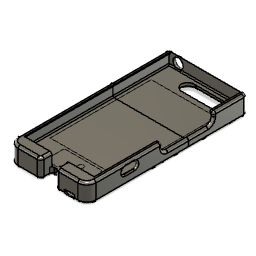
CoverMk5 v70 (Autodesk Fusion 360 design; units mm, degrees)
part number: BottomLid
Autodesk Fusion 360 part; units mm, degrees
(part 1 of 2)
sketch "Sketch1" plane through (0, 0, 0) normal (0, 1, 0) x (1, 0, 0) in component "BottomPart"
  line L0 (0, 0) -> (69, 0)
  line L1 (0, 0) -> (0, -90)
  line L2 (0, -90) -> (69, -90)
  line L3 (69, -90) -> (69, 0)
  line L4 (69, 0) -> (0, 0)
  line L5 (0, 0) -> (0, -90)
  dimension "d1" = 69
  dimension "d2" = 90
  constraint coincident L0.start L1.start
  constraint horizontal L0
  constraint perpendicular L0 L1
  constraint horizontal L2
  constraint vertical L3
  constraint horizontal L4
  constraint vertical L5
  measures "d1" distance of L0.start L0.end
  measures "d2" distance of L0.start L1.end
extrude "Extrude1" add sketch "Sketch1" along normal blind 0.5 makes body 1 in component "BottomPart"
sketch "Sketch2" plane through (0, 0.5, 0) normal (0, 1, 0) x (-1, 0, 0) in component "BottomPart"
  line L0 (0, 0) -> (0, 90)
  line L1 (0, 90) -> (-69, 90)
  line L2 (-69, 90) -> (-69, 0)
  line L3 (-69, 0) -> (0, 0)
  line L4 (0, 90) -> (-28, 90)
  line L5 (-69, 90) -> (-41, 90)
  line L6 (-41, 90) -> (-41, 80)
  line L7 (-41, 80) -> (-28, 80)
  line L8 (-28, 80) -> (-28, 90)
  line L9 (-28, 90) -> (-41, 90)
  line L10 (-41, 90) -> (-41, 80)
  dimension "d5" = 28
  dimension "d6" = 28
  dimension "d7" = 10
  constraint coincident L0.end L1.start
  constraint perpendicular L0 L4
  constraint coincident L1.end L2.start
  constraint perpendicular L2 L5
  constraint perpendicular L5 L6
  constraint horizontal L7
  constraint vertical L8
  constraint horizontal L9
  constraint vertical L10
  measures "d5" distance of L0.end L4.end
  measures "d6" distance of L1.end L5.end
  measures "d7" distance of L5.end L6.end
extrude "Extrude2" cut sketch "Sketch2" against normal blind 2 contours L1 L6 L7 L8 L9 L10 bodies 1 in component "BottomPart"
sketch "Sketch3" plane through (0, 0.5, 0) normal (0, 1, 0) x (-1, 0, 0) in component "BottomPart"
  line L0 (-41, 80) -> (-41, 90)
  line L1 (-41, 90) -> (-69, 90)
  line L2 (-69, 90) -> (-69, 0)
  line L3 (-69, 0) -> (0, 0)
  line L4 (0, 0) -> (0, 90)
  line L5 (0, 90) -> (-28, 90)
  line L6 (-28, 90) -> (-28, 80)
  line L7 (-28, 80) -> (-41, 80)
  line L8 (0, 0) -> (-2, 0)
  line L9 (-28, 80) -> (0, 80)
  line L10 (-2, 0) -> (-2, 80)
  line L11 (-41, 80) -> (-69, 80)
  line L12 (-69, 0) -> (-67, 0)
  line L13 (-67, 0) -> (-67, 80)
  dimension "d10" = 2
  dimension "d11" = 2
  constraint coincident L3.end L4.start
  constraint perpendicular L4 L8
  constraint coincident L6.end L7.start
  constraint coincident L4 L9.end
  constraint perpendicular L4 L9
  constraint coincident L9 L10.end
  constraint perpendicular L9 L10
  constraint coincident L0.start L7.end
  constraint coincident L2 L11.end
  constraint perpendicular L2 L11
  constraint coincident L2.end L3.start
  constraint perpendicular L2 L12
  constraint coincident L11 L13.end
  constraint perpendicular L11 L13
  measures "d10" distance of L3.end L8.end
  measures "d11" distance of L2.end L12.end
extrude "Extrude3" add sketch "Sketch3" along normal blind 10.5 contours L0 L1 L2 L11 | L4 L5 L6 L9 | L2 L3 L11 L12 L13 | L3 L4 L8 L9 L10 bodies 1 in component "BottomPart"
extrude "Extrude4" add 1 faces at (32.3333, 0, 26.6667) along direction (0, -1, 0) blind 4 on bodies 1 bodies 1 in component "BottomPart"
sketch "Sketch13" plane through (0, -4, 0) normal (0, -1, 0) x (1, 0, 0) in component "BottomPart"
  line L0 (41, 90) -> (41, 80)
  line L1 (41, 80) -> (28, 80)
  line L2 (28, 80) -> (28, 90)
  line L3 (28, 90) -> (0, 90)
  line L4 (0, 90) -> (0, 0)
  line L5 (0, 0) -> (69, 0)
  line L6 (69, 0) -> (69, 90)
  line L7 (69, 90) -> (41, 90)
  line L8 (0, 90) -> (2, 90)
  line L9 (2, 90) -> (2, 88)
  line L10 (2, 88) -> (0, 88)
  line L11 (0, 88) -> (0, 90)
  line L12 (28, 90) -> (26, 90)
  line L13 (26, 90) -> (26, 88)
  line L14 (26, 88) -> (28, 88)
  line L15 (28, 88) -> (28, 90)
  line L16 (28, 80) -> (26, 80)
  line L17 (26, 80) -> (26, 78)
  line L18 (26, 78) -> (28, 78)
  line L19 (28, 78) -> (28, 80)
  line L20 (41, 80) -> (43, 80)
  line L21 (43, 80) -> (43, 78)
  line L22 (43, 78) -> (41, 78)
  line L23 (41, 78) -> (41, 80)
  line L24 (41, 90) -> (43, 90)
  line L25 (43, 90) -> (43, 88)
  line L26 (43, 88) -> (41, 88)
  line L27 (41, 88) -> (41, 90)
  line L28 (69, 90) -> (67, 90)
  line L29 (67, 90) -> (67, 88)
  line L30 (67, 88) -> (69, 88)
  line L31 (69, 88) -> (69, 90)
  line L32 (69, 0) -> (67, 0)
  line L33 (0, 0) -> (2, 0)
  line L34 (2, 0) -> (2, 88)
  line L35 (26, 88) -> (2, 88)
  line L36 (26, 88) -> (26, 80)
  line L37 (28, 78) -> (41, 78)
  line L38 (43, 80) -> (43, 88)
  line L39 (43, 88) -> (67, 88)
  line L40 (67, 88) -> (67, 0)
  dimension "d181" = 2
  dimension "d182" = 2
  dimension "d183" = 2
  dimension "d184" = 2
  dimension "d185" = 2
  dimension "d186" = 2
  dimension "d187" = 2
  dimension "d188" = 2
  dimension "d189" = 2
  dimension "d190" = 2
  dimension "d191" = 2
  dimension "d192" = 2
  dimension "d193" = 2
  dimension "d194" = 2
  constraint horizontal L8
  constraint vertical L9
  constraint horizontal L10
  constraint vertical L11
  constraint coincident L3.end L4.start
  constraint horizontal L12
  constraint vertical L13
  constraint horizontal L14
  constraint vertical L15
  constraint coincident L2.end L3.start
  constraint horizontal L16
  constraint vertical L17
  constraint horizontal L18
  constraint vertical L19
  constraint coincident L1.end L2.start
  constraint horizontal L20
  constraint vertical L21
  constraint horizontal L22
  constraint vertical L23
  constraint coincident L0.end L1.start
  constraint horizontal L24
  constraint vertical L25
  constraint horizontal L26
  constraint vertical L27
  constraint coincident L0.start L7.end
  constraint horizontal L28
  constraint vertical L29
  constraint horizontal L30
  constraint vertical L31
  constraint coincident L6.end L7.start
  constraint coincident L5.end L6.start
  constraint perpendicular L6 L32
  constraint coincident L4.end L5.start
  constraint perpendicular L4 L33
  measures "d181" distance of L3.end L8.end
  measures "d182" distance of L3.end L10.end
  measures "d183" distance of L2.end L12.end
  measures "d184" distance of L2.end L14.end
  measures "d185" distance of L1.end L16.end
  measures "d186" distance of L1.end L18.end
  measures "d187" distance of L0.end L20.end
  measures "d188" distance of L0.end L22.end
  measures "d189" distance of L0.start L24.end
  measures "d190" distance of L0.start L26.end
  measures "d191" distance of L6.end L28.end
  measures "d192" distance of L6.end L30.end
  measures "d193" distance of L5.end L32.end
  measures "d194" distance of L4.end L33.end
extrude "Extrude19" cut sketch "Sketch13" against normal blind 4 contours L5 L17 L18 L21 L22 L34 L35 L36 L37 L38 L39 L40 bodies 1 in component "BottomPart"
sketch "Sketch4" plane through (0, 0, 0) normal (0, -1, 0) x (1, 0, 0) in component "BottomPart"
  line L0 (2, 88) -> (2, 2)
  line L1 (2, 2) -> (67, 2)
  line L2 (67, 2) -> (67, 88)
  line L3 (67, 88) -> (43, 88)
  line L4 (43, 88) -> (43, 78)
  line L5 (43, 78) -> (26, 78)
  line L6 (26, 78) -> (26, 88)
  line L7 (26, 88) -> (2, 88)
  line L8 (67, 88) -> (66, 88)
  line L9 (66, 88) -> (66, 82)
  line L10 (66, 82) -> (67, 82)
  line L11 (67, 82) -> (67, 88)
  circle A0 centre (66, 82) radius 0.95
  line L12 (66, 82) -> (64, 82)
  line L13 (64, 82) -> (64, 88)
  line L14 (64, 82) -> (67, 82)
  line L15 (67, 82) -> (67, 79)
  line L16 (67, 79) -> (64, 79)
  line L17 (64, 79) -> (64, 82)
  line L18 (43, 78) -> (39, 78)
  line L19 (39, 78) -> (39, 72)
  line L20 (39, 72) -> (43, 72)
  line L21 (43, 72) -> (43, 78)
  line L22 (41, 78) -> (41, 72)
  circle A1 centre (41, 75) radius 0.95
  line L23 (43, 88) -> (43, 78)
  line L24 (43, 78) -> (26, 78)
  line L25 (26, 78) -> (26, 88)
  line L26 (26, 88) -> (2, 88)
  line L27 (2, 88) -> (2, 0)
  line L28 (2, 0) -> (67, 0)
  line L29 (67, 0) -> (67, 88)
  line L30 (67, 88) -> (43, 88)
  dimension "d19" = 1
  dimension "d20" = 6
  dimension "d21" = 1.9
  dimension "d22" = 2
  dimension "d23" = 3
  dimension "d24" = 4
  dimension "d25" = 6
  dimension "d26" = 1.9
  constraint horizontal L8
  constraint vertical L9
  constraint horizontal L10
  constraint vertical L11
  constraint coincident L2.end L3.start
  constraint coincident L9.end L10.start
  constraint perpendicular L9 L12
  constraint coincident L3 L13.end
  constraint perpendicular L3 L13
  constraint horizontal L14
  constraint vertical L15
  constraint horizontal L16
  constraint vertical L17
  constraint horizontal L18
  constraint vertical L19
  constraint horizontal L20
  constraint vertical L21
  constraint coincident L4.end L5.start
  constraint midpoint L18 L22.start
  constraint midpoint L20 L22.end
  constraint midpoint L22 A1.centre
  measures "d19" distance of L2.end L8.end
  measures "d20" distance of L2.end L10.end
  measures "d21" diameter of A0
  measures "d22" distance of L9.end L12.end
  measures "d23" distance of L12.end L16.end
  measures "d24" distance of L4.end L18.end
  measures "d25" distance of L4.end L20.end
  measures "d26" diameter of A1
extrude "Extrude6" add sketch "Sketch4" along normal blind 4 contours L2 L10 A0 L12 L14 L15 L16 L17 L29 | L5 L18 L19 L20 L22 A1 L24 | L2 L3 L8 L9 L10 L11 A0 L14 L29 L30 | L5 L18 L20 L21 L22 A1 L24 | L3 L9 A0 L12 L13 L14 L30 bodies 1 in component "BottomPart"
sketch "Sketch5" plane through (0, -4, 0) normal (0, -1, 0) x (1, 0, 0) in component "BottomPart"
  line L0 (34.5, 80) -> (30.5, 80)
  line L1 (30.5, 80) -> (38.5, 80)
  line L2 (38.5, 80) -> (38.5, 78)
  line L3 (38.5, 78) -> (30.5, 78)
  line L4 (30.5, 78) -> (30.5, 80)
  line L5 (67, 79) -> (67, 0)
  line L6 (67, 0) -> (69, 0)
  line L7 (69, 0) -> (69, 90)
  line L8 (69, 90) -> (41, 90)
  line L9 (41, 90) -> (41, 80)
  line L10 (41, 80) -> (28, 80)
  line L11 (28, 80) -> (28, 90)
  line L12 (28, 90) -> (0, 90)
  line L13 (0, 90) -> (0, 0)
  line L14 (0, 0) -> (2, 0)
  line L15 (2, 0) -> (2, 88)
  line L16 (2, 88) -> (26, 88)
  line L17 (26, 88) -> (26, 78)
  line L18 (26, 78) -> (39, 78)
  line L19 (43, 72) -> (43, 88)
  line L20 (43, 88) -> (64, 88)
  circle A0 centre (41, 75) radius 0.95
  line L21 (39, 78) -> (39, 72)
  line L22 (39, 72) -> (43, 72)
  line L23 (64, 88) -> (64, 79)
  line L24 (64, 79) -> (67, 79)
  circle A1 centre (66, 82) radius 0.95
  dimension "d29" = 4
  dimension "d30" = 8
  constraint horizontal L1
  constraint vertical L2
  constraint horizontal L3
  constraint vertical L4
  measures "d29" distance of L0.start L0.end
  measures "d30" distance of L0.end L1.end
extrude "Extrude7" cut sketch "Sketch5" against normal blind 2.5 contours L0 L1 L2 L3 L4 L10 L18 bodies 1 in component "BottomPart"
sketch "Sketch6" plane through (0, 0, 0) normal (0, -1, 0) x (1, 0, 0) in component "BottomPart"
  line L0 (43, 88) -> (64, 88)
  line L1 (64, 88) -> (64, 61)
  line L2 (64, 61) -> (43, 61)
  line L3 (43, 61) -> (43, 88)
  line L4 (64, 61) -> (67, 61)
  line L5 (64, 61) -> (64, 60)
  line L6 (64, 60) -> (2, 60)
  line L7 (2, 60) -> (2, 61)
  line L8 (2, 61) -> (64, 61)
  line L9 (64, 61) -> (64, 60)
  line L10 (43, 72) -> (39, 72)
  line L11 (39, 72) -> (39, 65)
  line L12 (39, 65) -> (43, 65)
  line L13 (43, 65) -> (43, 72)
  line L14 (26, 78) -> (20, 78)
  line L15 (20, 78) -> (20, 61)
  line L16 (64, 61) -> (67, 61)
  line L17 (67, 61) -> (67, 65)
  line L18 (67, 65) -> (64, 65)
  line L19 (64, 65) -> (64, 61)
  line L20 (30.5, 78) -> (38.5, 78)
  line L21 (38.5, 78) -> (38.5, 80)
  line L22 (38.5, 80) -> (30.5, 80)
  line L23 (30.5, 80) -> (30.5, 78)
  line L24 (39, 72) -> (39, 78)
  line L25 (39, 78) -> (26, 78)
  line L26 (26, 78) -> (26, 88)
  line L27 (26, 88) -> (2, 88)
  line L28 (2, 88) -> (2, 0)
  line L29 (2, 0) -> (67, 0)
  line L30 (67, 0) -> (67, 79)
  line L31 (67, 79) -> (64, 79)
  line L32 (64, 79) -> (64, 88)
  line L33 (64, 88) -> (43, 88)
  line L34 (43, 88) -> (43, 72)
  line L35 (43, 72) -> (39, 72)
  dimension "d33" = 21
  dimension "d34" = 27
  dimension "d35" = 1
  dimension "d36" = 1
  dimension "d37" = 4
  dimension "d38" = 7
  dimension "d39" = 6
  dimension "d42" = 4
  constraint horizontal L0
  constraint vertical L1
  constraint horizontal L2
  constraint vertical L3
  constraint perpendicular L2 L5
  constraint horizontal L6
  constraint vertical L7
  constraint horizontal L8
  constraint vertical L9
  constraint horizontal L10
  constraint vertical L11
  constraint horizontal L12
  constraint vertical L13
  constraint coincident L8 L15.end
  constraint perpendicular L8 L15
  constraint horizontal L16
  constraint vertical L17
  constraint horizontal L18
  constraint vertical L19
  measures "d33" distance of L0.start L0.end
  measures "d34" distance of L0.start L2.end
  measures "d35" distance of L1.end L5.end
  measures "d36" distance of L5.end L1.end
  measures "d37" distance of L10.start L10.end
  measures "d38" distance of L10.start L12.end
  measures "d39" distance of L14.start L14.end
  measures "d42" distance of L1.end L18.end
extrude "Extrude8" add sketch "Sketch6" along normal blind 4 contours L3 L10 L11 L12 L13 L35 | L1 L18 L30 L31 | L2 L5 L6 L7 L8 L9 L28 | L8 L14 L15 L26 L27 L28 bodies 1 in component "BottomPart"
sketch "Sketch7" plane through (0, -4, 0) normal (0, -1, 0) x (1, 0, 0) in component "BottomPart"
  line L0 (0, 90) -> (3, 90)
  line L1 (3, 90) -> (3, 82)
  line L2 (3, 82) -> (0, 82)
  line L3 (0, 82) -> (0, 90)
  circle A0 centre (3, 82) radius 0.95
  line L4 (41, 80) -> (38.5, 80)
  line L5 (69, 90) -> (41, 90)
  line L6 (67, 0) -> (69, 0)
  line L7 (38.5, 78) -> (39, 78)
  circle A1 centre (66, 82) radius 0.95
  line L8 (38.5, 80) -> (38.5, 78)
  line L9 (39, 78) -> (39, 65)
  line L10 (43, 65) -> (43, 88)
  line L11 (43, 88) -> (64, 88)
  line L12 (64, 88) -> (64, 65)
  line L13 (67, 65) -> (67, 0)
  line L14 (69, 0) -> (69, 90)
  line L15 (41, 90) -> (41, 80)
  circle A2 centre (41, 75) radius 0.95
  line L16 (39, 65) -> (43, 65)
  line L17 (64, 65) -> (67, 65)
  dimension "d43" = 3
  dimension "d44" = 8
  dimension "d45" = 1.9
  constraint horizontal L0
  constraint vertical L1
  constraint horizontal L2
  constraint vertical L3
  constraint coincident L1.end L2.start
  measures "d43" distance of L0.start L0.end
  measures "d44" distance of L0.start L2.end
  measures "d45" diameter of A0
extrude "Extrude9" cut sketch "Sketch7" against normal blind 2.5 contours L1 L2 A0 | L1 L2 A0 bodies 1 in component "BottomPart"
sketch "Sketch8" plane through (0, -4, 0) normal (0, -1, 0) x (1, 0, 0) in component "BottomPart"
  line L0 (67, 2) -> (67, 0)
  line L1 (2, 2) -> (2, 0)
  line L2 (41, 80) -> (38.5, 80)
  line L3 (69, 90) -> (41, 90)
  line L4 (67, 0) -> (69, 0)
  line L5 (38.5, 78) -> (39, 78)
  circle A0 centre (66, 82) radius 0.95
  line L6 (38.5, 80) -> (38.5, 78)
  line L7 (39, 78) -> (39, 65)
  line L8 (39, 65) -> (43, 65)
  line L9 (43, 65) -> (43, 88)
  line L10 (43, 88) -> (64, 88)
  line L11 (64, 88) -> (64, 65)
  line L12 (64, 65) -> (67, 65)
  line L13 (67, 65) -> (67, 0)
  line L14 (69, 0) -> (69, 90)
  line L15 (41, 90) -> (41, 80)
  circle A1 centre (41, 75) radius 0.95
sketch "Sketch9" plane through (0, 0, 0) normal (0, -1, 0) x (1, 0, 0) in component "BottomPart"
  line L0 (2, 0) -> (2, 10)
  line L1 (67, 0) -> (67, 10)
  line L2 (2, 10) -> (2.25, 10)
  circle A0 centre (2.25, 10) radius 0.95
  line L3 (67, 10) -> (66.75, 10)
  circle A1 centre (66.75, 10) radius 0.95
  line L4 (67, 10) -> (67, 14)
  line L5 (67, 14) -> (64.5, 14)
  line L6 (67, 10) -> (67, 6)
  line L7 (67, 6) -> (64.5, 6)
  line L8 (64.5, 6) -> (64.5, 14)
  line L9 (64.5, 14) -> (67, 14)
  line L10 (67, 14) -> (67, 6)
  line L11 (2, 10) -> (2, 14)
  line L12 (2, 14) -> (4.5, 14)
  line L13 (2, 10) -> (2, 6)
  line L14 (2, 6) -> (4.5, 6)
  line L15 (4.5, 6) -> (4.5, 14)
  line L16 (4.5, 14) -> (2, 14)
  line L17 (2, 14) -> (2, 6)
  line L18 (2, 10) -> (2, 30)
  line L19 (67, 10) -> (67, 30)
  line L20 (2, 30) -> (2.25, 30)
  circle A2 centre (2.25, 30) radius 0.95
  line L21 (67, 30) -> (66.75, 30)
  circle A3 centre (66.75, 30) radius 0.95
  line L22 (67, 30) -> (67, 34)
  line L23 (67, 30) -> (67, 26)
  line L24 (67, 34) -> (64.5, 34)
  line L25 (64.5, 34) -> (67, 34)
  line L26 (67, 34) -> (67, 26)
  line L27 (67, 26) -> (64.5, 26)
  line L28 (64.5, 26) -> (64.5, 34)
  line L29 (2, 30) -> (2, 34)
  line L30 (2, 30) -> (2, 26)
  line L31 (2, 34) -> (4.5, 34)
  line L32 (2, 26) -> (4.5, 26)
  line L33 (4.5, 26) -> (4.5, 34)
  line L34 (4.5, 34) -> (2, 34)
  line L35 (2, 34) -> (2, 26)
  line L36 (28, 80) -> (28, 90)
  line L37 (28, 90) -> (0, 90)
  line L38 (0, 90) -> (0, 0)
  line L39 (0, 0) -> (67, 0)
  line L40 (43, 88) -> (43, 65)
  line L41 (43, 65) -> (39, 65)
  line L42 (39, 65) -> (39, 78)
  line L43 (39, 78) -> (30.5, 78)
  line L44 (30.5, 78) -> (30.5, 80)
  line L45 (30.5, 80) -> (28, 80)
  line L46 (67, 0) -> (67, 84)
  line L47 (67, 84) -> (64, 84)
  line L48 (64, 84) -> (64, 88)
  line L49 (64, 88) -> (43, 88)
  line L50 (43, 88) -> (43, 65)
  line L51 (43, 65) -> (39, 65)
  line L52 (39, 65) -> (39, 78)
  line L53 (39, 78) -> (20, 78)
  line L54 (2, 0) -> (67, 0)
  line L55 (67, 0) -> (67, 65)
  line L56 (64, 65) -> (64, 88)
  line L57 (64, 88) -> (43, 88)
  line L58 (20, 78) -> (20, 61)
  line L59 (20, 61) -> (64, 61)
  line L60 (64, 61) -> (64, 60)
  line L61 (64, 60) -> (2, 60)
  line L62 (2, 60) -> (2, 0)
  line L63 (67, 65) -> (64, 65)
  dimension "d50" = 10
  dimension "d51" = 10
  dimension "d52" = 0.25
  dimension "d53" = 1.9
  dimension "d54" = 0.25
  dimension "d55" = 1.9
  dimension "d56" = 4
  dimension "d57" = 2.5
  dimension "d58" = 4
  dimension "d59" = 4
  dimension "d60" = 2.5
  dimension "d61" = 4
  dimension "d66" = 20
  dimension "d67" = 20
  dimension "d68" = 0.25
  dimension "d69" = 1.9
  dimension "d70" = 0.25
  dimension "d71" = 1.9
  dimension "d72" = 4
  dimension "d73" = 4
  dimension "d74" = 2.5
  dimension "d75" = 4
  dimension "d76" = 4
  dimension "d77" = 2.5
  constraint horizontal L2
  constraint coincident L2.end A0.centre
  constraint perpendicular L1 L3
  constraint coincident L3.end A1.centre
  constraint perpendicular L3 L4
  constraint perpendicular L4 L5
  constraint perpendicular L3 L6
  constraint horizontal L7
  constraint vertical L8
  constraint horizontal L9
  constraint vertical L10
  constraint perpendicular L2 L11
  constraint perpendicular L11 L12
  constraint perpendicular L2 L13
  constraint horizontal L14
  constraint vertical L15
  constraint horizontal L16
  constraint vertical L17
  constraint perpendicular L16 L18
  constraint perpendicular L3 L19
  constraint perpendicular L18 L20
  constraint coincident L20.end A2.centre
  constraint perpendicular L19 L21
  constraint coincident L21.end A3.centre
  constraint perpendicular L21 L22
  constraint perpendicular L21 L23
  constraint perpendicular L22 L24
  constraint horizontal L25
  constraint vertical L26
  constraint horizontal L27
  constraint vertical L28
  constraint perpendicular L20 L29
  constraint perpendicular L20 L30
  constraint perpendicular L29 L31
  constraint horizontal L32
  constraint vertical L33
  constraint horizontal L34
  constraint vertical L35
  constraint coincident L0.start L54.start
  constraint coincident L29.end L62
  measures "d50" distance of L0.end L0.start
  measures "d51" distance of L1.start L1.end
  measures "d52" distance of L0.end L2.end
  measures "d53" diameter of A0
  measures "d54" distance of L1.end L3.end
  measures "d55" diameter of A1
  measures "d56" distance of L1.end L4.end
  measures "d57" distance of L4.end L5.end
  measures "d58" distance of L1.end L6.end
  measures "d59" distance of L0.end L11.end
  measures "d60" distance of L11.end L12.end
  measures "d61" distance of L0.end L13.end
  measures "d66" distance of L0.end L18.end
  measures "d67" distance of L1.end L19.end
  measures "d68" distance of L18.end L20.end
  measures "d69" diameter of A2
  measures "d70" distance of L19.end L21.end
  measures "d71" diameter of A3
  measures "d72" distance of L19.end L22.end
  measures "d73" distance of L19.end L23.end
  measures "d74" distance of L22.end L24.end
  measures "d75" distance of L18.end L29.end
  measures "d76" distance of L18.end L30.end
  measures "d77" distance of L31.end L29.end
extrude "Extrude11" cut sketch "Sketch9" along normal blind 4 contours L0 A0 L11 L13 L17 L18 L62 | L0 A0 L11 L13 L17 L18 L62 | L1 A1 L4 L6 L10 L19 L46 L55 | L1 A1 L4 L6 L10 L19 L46 L55 | L18 A2 L29 L30 L35 L62 | L18 A2 L29 L30 L35 L62 | L19 A3 L22 L23 L26 L46 L55 | L19 A3 L22 L23 L26 L46 L55 bodies 1 in component "BottomPart"
extrude "Extrude12" add sketch "Sketch9" along normal blind 4 contours L0 A0 L11 L12 L13 L14 L15 L16 L17 L18 L62 | L1 A1 L4 L5 L6 L7 L8 L9 L10 L19 L46 L55 | L18 A2 L29 L30 L31 L32 L33 L34 L35 L62 | L19 A3 L22 L23 L24 L25 L26 L27 L28 L46 L55 bodies 1 in component "BottomPart"
sketch "Sketch10" plane through (0, 0, 0) normal (0, 0, -1) x (-1, 0, 0) in component "BottomPart"
  line L0 (0, -4) -> (0, 11)
  line L1 (0, 11) -> (-2, 11)
  line L2 (-2, 11) -> (-2, 0.5)
  line L3 (-2, 0.5) -> (-67, 0.5)
  line L4 (-67, 0.5) -> (-67, 11)
  line L5 (-67, 11) -> (-69, 11)
  line L6 (-69, 11) -> (-69, -4)
  line L7 (-2, 11) -> (-3.5, 11)
  line L8 (-3.5, 11) -> (-3.5, 10)
  line L9 (-3.5, 10) -> (-2, 10)
  line L10 (-2, 10) -> (-2, 11)
  line L11 (-67, 11) -> (-65.5, 11)
  line L12 (-65.5, 11) -> (-65.5, 10)
  line L13 (-65.5, 10) -> (-67, 10)
  line L14 (-67, 10) -> (-67, 11)
  line L15 (-67, 0) -> (-2, 0)
  line L16 (-2, -4) -> (0, -4)
  line L17 (-67, -4) -> (-67, 0)
  line L18 (-2, 0) -> (-2, -4)
  line L19 (-69, -4) -> (-67, -4)
  dimension "d78" = 1.5
  dimension "d79" = 1
  dimension "d80" = 1.5
  dimension "d81" = 1
  constraint horizontal L7
  constraint vertical L8
  constraint horizontal L9
  constraint vertical L10
  constraint coincident L1.end L2.start
  constraint horizontal L11
  constraint vertical L12
  constraint horizontal L13
  constraint vertical L14
  constraint coincident L4.end L5.start
  measures "d78" distance of L1.end L7.end
  measures "d79" distance of L1.end L9.end
  measures "d80" distance of L4.end L11.end
  measures "d81" distance of L4.end L13.end
extrude "Extrude13" add sketch "Sketch10" against normal blind 80 contours L2 L7 L8 L9 L10 | L4 L11 L12 L13 L14 bodies 1 in component "BottomPart"
sketch "Sketch11" plane through (67, 0, 0) normal (-1, 0, 0) x (0, 0, 1) in component "BottomPart"
  line L0 (80, 10) -> (0, 10)
  line L1 (0, 10) -> (0, 0.5)
  line L2 (0, 0.5) -> (80, 0.5)
  line L3 (80, 0.5) -> (80, 10)
  line L4 (80, 0.5) -> (80, 2.25)
  line L5 (80, 2.25) -> (23.5, 2.25)
  line L6 (23.5, 2.25) -> (0, 2.25)
  line L7 (0, 2.25) -> (0, 12.25)
  line L8 (0, 12.25) -> (23.5, 12.25)
  line L9 (23.5, 12.25) -> (23.5, 2.25)
  dimension "d84" = 1.75
  dimension "d85" = 56.5
  dimension "d86" = 23.5
  dimension "d87" = 10
  constraint coincident L2.end L3.start
  constraint perpendicular L2 L4
  constraint perpendicular L4 L5
  constraint horizontal L6
  constraint vertical L7
  constraint horizontal L8
  constraint vertical L9
  measures "d84" distance of L2.end L4.end
  measures "d85" distance of L4.end L5.end
  measures "d86" distance of L5.end L6.end
  measures "d87" distance of L5.end L8.end
extrude "Extrude1'" add 1 faces at (0.6667, 2.5, 0) along direction (0, 0, -1) blind 49.75 separate body on bodies 1 makes body 2 in component "TopPart"
sketch "Sketch1 (2)" plane through (0, 0, -49.75) normal (0, 0, -1) x (-1, 0, 0) in component "TopPart"
  line L0 (0, -4) -> (0, 11)
  line L1 (0, 11) -> (-3.5, 11)
  line L2 (-3.5, 11) -> (-3.5, 10)
  line L3 (-3.5, 10) -> (-2, 10)
  line L4 (-2, 10) -> (-2, 0.5)
  line L5 (-2, 0.5) -> (-67, 0.5)
  line L6 (-67, 0.5) -> (-67, 10)
  line L7 (-67, 10) -> (-65.5, 10)
  line L8 (-65.5, 10) -> (-65.5, 11)
  line L9 (-65.5, 11) -> (-69, 11)
  line L10 (-69, 11) -> (-69, -4)
  line L11 (-2, -4) -> (-67, -4)
  line L12 (-65.5, 11) -> (-3.5, 11)
  line L13 (-69, -4) -> (-67, -4)
  line L14 (-67, 0) -> (-2, 0)
  line L15 (-67, -4) -> (-67, 0)
  line L16 (-2, 0) -> (-2, -4)
  line L17 (-2, -4) -> (0, -4)
  constraint coincident L8.end L9.start
  constraint coincident L1.end L2.start
  constraint coincident L11.end L13.end
  constraint coincident L11.start L16.end
extrude "Extrude2'" add sketch "Sketch1 (2)" along normal blind 2 bodies 2 in component "TopPart"
sketch "Sketch2 (2)" plane through (0, 0, 0) normal (0, -1, 0) x (1, 0, 0) in component "TopPart"
  line L0 (2, 0) -> (0, 0)
  line L1 (0, 0) -> (0, -30)
  line L2 (0, -30) -> (67, -30)
  line L3 (0, 0) -> (0, -51.75)
  line L4 (0, -51.75) -> (2, -51.75)
  line L5 (2, -51.75) -> (2, 0)
  line L6 (67, 0) -> (2, 0)
  line L7 (2, 0) -> (2, -49.75)
  line L8 (2, -49.75) -> (67, -49.75)
  line L9 (67, -49.75) -> (67, 0)
  line L10 (67, 0) -> (2, 0)
  line L11 (2, 0) -> (2, -49.75)
  line L12 (2, -49.75) -> (67, -49.75)
  line L13 (67, -49.75) -> (67, 0)
  dimension "d92" = 30
  constraint coincident L0.end L1.start
  constraint perpendicular L0 L1
  constraint coincident L2.end L9
  constraint perpendicular L2 L9
  measures "d92" distance of L0.end L1.end
extrude "Extrude3'" add sketch "Sketch2 (2)" along normal blind 4 contours L2 L5 L7 L8 L9 L11 L12 L13 bodies 2 in component "TopPart"
sketch "Sketch2 (3)" plane through (0, 0, 0) normal (0, -1, 0) x (1, 0, 0)
  line L0 (67, 0) -> (2, 0)
  line L1 (2, 0) -> (2, -30)
  line L2 (67, -30) -> (67, 0)
  line L3 (2, 0) -> (67, 0)
  line L4 (67, 0) -> (67, -30)
  line L5 (67, -30) -> (2, -30)
  line L6 (2, -30) -> (2, 0)
  line L7 (2, -30) -> (67, -30)
  dimension "d199" = 30
  constraint horizontal L3
  constraint vertical L4
  constraint horizontal L5
  constraint vertical L6
  constraint coincident L0.end L1.start
  measures "d199" distance of L0.end L1.end
sketch "Sketch3 (2)" plane through (0, 0, 0) normal (0, -1, 0) x (1, 0, 0)
  line L0 (67, -30) -> (67, 0)
  line L1 (67, 0) -> (2, 0)
  line L2 (2, 0) -> (2, -30)
  line L3 (2, -15) -> (2.25, -15)
  line L4 (67, -15) -> (66.75, -15)
  circle A0 centre (2.25, -15) radius 0.95
  circle A1 centre (66.75, -15) radius 0.95
  line L5 (67, -15) -> (67, -11)
  line L6 (67, -11) -> (64.5, -11)
  line L7 (64.5, -11) -> (64.5, -19)
  line L8 (64.5, -19) -> (67, -19)
  line L9 (67, -19) -> (67, -11)
  line L10 (2, -15) -> (2, -11)
  line L11 (2, -11) -> (4.5, -11)
  line L12 (4.5, -11) -> (4.5, -19)
  line L13 (4.5, -19) -> (2, -19)
  line L14 (2, -19) -> (2, -11)
  line L15 (2, -30) -> (67, -30)
  dimension "d202" = 0.25
  dimension "d203" = 0.25
  dimension "d204" = 1.9
  dimension "d205" = 1.9
  dimension "d206" = 4
  dimension "d207" = 2.5
  dimension "d208" = 8
  dimension "d209" = 4
  dimension "d210" = 2.5
  dimension "d211" = 8
  constraint midpoint L2 L3.start
  constraint horizontal L3
  constraint midpoint L0 L4.start
  constraint horizontal L4
  constraint coincident L3.end A0.centre
  constraint coincident L4.end A1.centre
  constraint perpendicular L4 L5
  constraint horizontal L6
  constraint vertical L7
  constraint horizontal L8
  constraint vertical L9
  constraint perpendicular L3 L10
  constraint horizontal L11
  constraint vertical L12
  constraint horizontal L13
  constraint vertical L14
  measures "d202" distance of L3.start L3.end
  measures "d203" distance of L4.start L4.end
  measures "d204" diameter of A0
  measures "d205" diameter of A1
  measures "d206" distance of L4.start L5.end
  measures "d207" distance of L5.end L6.end
  measures "d208" distance of L5.end L8.end
  measures "d209" distance of L3.start L10.end
  measures "d210" distance of L10.end L11.end
  measures "d211" distance of L10.end L13.end
extrude "Extrude11'" cut sketch "Sketch3 (2)" along normal blind 4 contours L0 A1 L5 L9 | L0 A1 L5 L9 | L2 A0 L10 L14 | L2 A0 L10 L14 bodies 2 in component "TopPart"
extrude "Extrude12'" add sketch "Sketch3 (2)" along normal blind 4 contours L0 A1 L5 L6 L7 L8 L9 | L2 A0 L10 L11 L12 L13 L14 bodies 2 in component "TopPart"
sketch "Sketch4 (2)" plane through (0, 0.5, 0) normal (0, 1, 0) x (-1, 0, 0) in component "TopPart"
  line L0 (-2, 0) -> (-67, 0)
  line L1 (-67, 0) -> (-67, -49.75)
  line L2 (-67, -49.75) -> (-2, -49.75)
  line L3 (-2, -49.75) -> (-2, 0)
  line L4 (-67, -49.75) -> (-58, -49.75)
  line L5 (-58, -49.75) -> (-58, -40.25)
  line L6 (-58, -40.25) -> (-67, -40.25)
  line L7 (-67, -40.25) -> (-67, -49.75)
  line L8 (-58, -40.25) -> (-28, -40.25)
  circle A0 centre (-58, -40.25) radius 5.5
  circle A1 centre (-28, -40.25) radius 5.5
  line L9 (-28, -45.75) -> (-58, -45.75)
  line L10 (-58, -45.75) -> (-58, -34.75)
  line L11 (-58, -34.75) -> (-28, -34.75)
  line L12 (-28, -34.75) -> (-28, -45.75)
  dimension "d111" = 9
  dimension "d112" = 9.5
  dimension "d113" = 30
  dimension "d114" = 11
  dimension "d115" = 11
  constraint horizontal L4
  constraint vertical L5
  constraint horizontal L6
  constraint vertical L7
  constraint coincident L1.end L2.start
  constraint perpendicular L5 L8
  constraint coincident L5.end L6.start
  constraint coincident L8.end A1.centre
  constraint horizontal L9
  constraint vertical L10
  constraint horizontal L11
  constraint vertical L12
  constraint coincident A0 L10.end
  constraint coincident A1 L9.start
  measures "d111" distance of L1.end L4.end
  measures "d112" distance of L1.end L6.end
  measures "d113" distance of L5.end L8.end
  measures "d114" diameter of A0
  measures "d115" diameter of A1
extrude "Extrude6'" cut sketch "Sketch4 (2)" against normal blind 6 contours L6 A0 L10 | L5 L6 A0 L10 | L5 L8 A0 L10 | L8 A0 A1 L9 | L8 A0 L10 | L8 A0 A1 L11 | A1 L12 | L8 A1 L12 | L8 A1 L12 bodies 2 in component "TopPart"
draft "Draft1" angle -30 neutral plane through (2, 0.5, 0) pull (0, 1, 0) 4 faces at (24.4647, -1, -36.0368) (48, -2.5, -34.75) (60.6304, -2.5, -35.4198) (38, -2.5, -45.75) on bodies 2 in component "TopPart"
sketch "Sketch5 (2)" plane through (0, -4, 0) normal (0, -1, 0) x (1, 0, 0) in component "TopPart"
  line L0 (2, -51.75) -> (12, -51.75)
  line L1 (12, -51.75) -> (12, -41.75)
  line L2 (12, -41.75) -> (2, -41.75)
  line L3 (2, -41.75) -> (2, -51.75)
  circle A0 centre (12, -41.75) radius 0.95
  line L4 (2, -30) -> (2, -19)
  line L5 (2, 0) -> (0, 0)
  line L6 (0, 0) -> (0, -51.75)
  line L7 (0, -51.75) -> (69, -51.75)
  line L8 (69, -51.75) -> (69, 0)
  line L9 (69, 0) -> (67, 0)
  line L10 (67, 0) -> (67, -11)
  line L11 (28, -32.1519) -> (58, -32.1519)
  arc A1 (58, -48.3481) -> (58, -32.1519) centre (58, -40.25) ccw
  line L12 (58, -48.3481) -> (28, -48.3481)
  arc A2 (28, -32.1519) -> (28, -48.3481) centre (28, -40.25) ccw
  circle A3 centre (66.75, -15) radius 0.95
  line L13 (67, -11) -> (64.5, -11)
  line L14 (64.5, -11) -> (64.5, -19)
  line L15 (64.5, -19) -> (67, -19)
  line L16 (67, -19) -> (67, -30)
  line L17 (4.5, -19) -> (4.5, -11)
  line L18 (2, -19) -> (4.5, -19)
  line L19 (4.5, -11) -> (2, -11)
  line L20 (2, -11) -> (2, 0)
  circle A4 centre (2.25, -15) radius 0.95
  line L21 (67, -30) -> (2, -30)
  dimension "d120" = 10
  dimension "d121" = 10
  dimension "d122" = 1.9
  constraint horizontal L0
  constraint vertical L1
  constraint horizontal L2
  constraint vertical L3
  constraint coincident L1.end L2.start
  measures "d120" distance of L0.start L0.end
  measures "d121" distance of L0.start L2.end
  measures "d122" diameter of A0
extrude "Extrude7'" cut sketch "Sketch5 (2)" against normal blind 2.5 contours L1 L2 A0 | L1 L2 A0 bodies 2 in component "TopPart"
extrude "Extrude14" cut sketch "Sketch11" along normal blind 1.5 contours L0 L1 L6 L7 L9 | L0 L7 L8 L9 bodies 1 in component "BottomPart"
extrude "Extrude15" cut sketch "Sketch11" against normal blind 2 contours L0 L1 L6 L7 L9 | L0 L7 L8 L9 bodies 1 in component "BottomPart"
sketch "Sketch6 (2)" plane through (67, 0, 0) normal (-1, 0, 0) x (0, 0, 1) in component "TopPart"
  line L0 (0, 0.5) -> (0, 10)
  line L1 (0, 10) -> (-49.75, 10)
  line L2 (-49.75, 10) -> (-49.75, 0.5)
  line L3 (-49.75, 0.5) -> (0, 0.5)
  line L4 (0, 0.5) -> (0, 2.25)
  line L5 (0, 2.25) -> (-22, 2.25)
  line L6 (-22, 2.25) -> (0, 2.25)
  line L7 (0, 2.25) -> (0, 14.25)
  line L8 (0, 14.25) -> (-22, 14.25)
  line L9 (-22, 14.25) -> (-22, 2.25)
  dimension "d129" = 1.75
  dimension "d130" = 22
  dimension "d131" = 12
  constraint coincident L0.start L3.end
  constraint perpendicular L3 L4
  constraint perpendicular L4 L5
  constraint horizontal L6
  constraint vertical L7
  constraint horizontal L8
  constraint vertical L9
  measures "d129" distance of L0.start L4.end
  measures "d130" distance of L4.end L5.end
  measures "d131" distance of L5.end L8.end
extrude "Extrude8'" cut sketch "Sketch6 (2)" along normal blind 2 contours L0 L1 L5 L6 L7 L9 | L1 L7 L8 L9 bodies 2 in component "TopPart"
extrude "Extrude9'" cut sketch "Sketch6 (2)" against normal blind 2 contours L0 L1 L5 L6 L7 L9 | L1 L7 L8 L9 bodies 2 in component "TopPart"
fillet "Fillet1" radius 1.5 2 edges at (2, 10, 40) (67, 10, 51.75) on bodies 1 in component "BottomPart"
fillet "Fillet1'" radius 1.5 2 edges at (2, 10, -24.875) (67, 10, -35.875) on bodies 2 in component "TopPart"
extrude "Extrude21" cut 1 faces at (33.1667, -1.5, 78.6667) along direction (0, 1, 0) blind 1.5 on bodies 1 bodies 1 in component "BottomPart"
sketch "Sketch14" plane through (0, 0, 88) normal (0, 0, -1) x (-1, 0, 0) in component "BottomPart"
  line L0 (-64, 0) -> (-64, -4)
  line L1 (-64, -4) -> (-43, -4)
  line L2 (-43, -4) -> (-43, 0)
  line L3 (-43, 0) -> (-64, 0)
  line L4 (-53.5, 0) -> (-53.5, -1.5)
  line L5 (-53.5, -1.5) -> (-58.1, -1.5)
  line L6 (-58.1, -1.5) -> (-48.9, -1.5)
  line L7 (-48.9, -1.5) -> (-48.9, -4)
  line L8 (-48.9, -4) -> (-58.1, -4)
  line L9 (-58.1, -4) -> (-58.1, -1.5)
  dimension "d218" = 1.5
  dimension "d219" = 4.6
  dimension "d220" = 9.2
  constraint midpoint L3 L4.start
  constraint perpendicular L3 L4
  constraint perpendicular L4 L5
  constraint horizontal L6
  constraint vertical L7
  constraint horizontal L8
  constraint vertical L9
  measures "d218" distance of L4.start L4.end
  measures "d219" distance of L4.end L5.end
  measures "d220" distance of L5.end L6.end
extrude "Extrude22" cut sketch "Sketch14" against normal blind 2 contours L1 L5 L6 L7 L8 L9 bodies 1 in component "BottomPart"
sketch "Sketch1 (3)" plane through (0, -4, 0) normal (0, -1, 0) x (1, 0, 0) in component "BottomLid"
  line L0 (2, 34) -> (2, 60)
  line L1 (2, 60) -> (64, 60)
  line L2 (64, 60) -> (64, 61)
  line L3 (64, 61) -> (20, 61)
  line L4 (20, 61) -> (20, 78)
  line L5 (20, 78) -> (30.5, 78)
  line L6 (30.5, 78) -> (30.5, 80)
  line L7 (30.5, 80) -> (28, 80)
  line L8 (28, 80) -> (28, 90)
  line L9 (28, 90) -> (0, 90)
  line L10 (0, 90) -> (0, 0)
  line L11 (0, 0) -> (2, 0)
  line L12 (2, 0) -> (2, 6)
  circle A0 centre (3, 82) radius 0.95
  line L13 (2, 0) -> (69, 0)
  line L14 (69, 0) -> (69, 90)
  line L15 (69, 90) -> (41, 90)
  line L16 (41, 90) -> (41, 80)
  line L17 (41, 80) -> (30.5, 80)
  line L18 (2.25, 30) -> (66.75, 30)
  line L19 (41, 80) -> (41, 75)
  line L20 (69, 90) -> (66, 90)
  line L21 (66, 90) -> (66, 82)
  line L22 (66, 82) -> (69, 82)
  line L23 (69, 82) -> (69, 90)
  circle A1 centre (66, 82) radius 0.95
  circle A2 centre (41, 75) radius 0.95
  circle A3 centre (66.75, 30) radius 0.95
  line L24 (2, 22.5) -> (69, 22.5)
  line L25 (2, 22.5) -> (0, 22.5)
  circle A4 centre (2.25, 30) radius 0.95
  line L26 (2, 6) -> (4.5, 6)
  line L27 (4.5, 6) -> (4.5, 14)
  line L28 (4.5, 14) -> (2, 14)
  line L29 (2, 14) -> (2, 26)
  line L30 (2, 26) -> (4.5, 26)
  line L31 (4.5, 26) -> (4.5, 34)
  line L32 (4.5, 34) -> (2, 34)
  circle A5 centre (2.25, 10) radius 0.95
  circle A6 centre (2.25, 30) radius 0.95
  dimension "d224" = 90
  dimension "d225" = 28
  dimension "d226" = 10
  dimension "d228" = 64.5
  dimension "d229" = 5
  dimension "d230" = 3
  dimension "d231" = 8
  dimension "d232" = 1.9
  dimension "d233" = 1.9
  dimension "d234" = 1.9
  dimension "d236" = 1.9
  constraint coincident L11.end L12.start
  constraint perpendicular L12 L13
  constraint perpendicular L13 L14
  constraint perpendicular L14 L15
  constraint perpendicular L15 L16
  constraint coincident L6.end L7.start
  constraint horizontal L18
  constraint perpendicular L17 L19
  constraint horizontal L20
  constraint vertical L21
  constraint horizontal L22
  constraint vertical L23
  constraint coincident L21.end L22.start
  constraint coincident L19.end A2.centre
  constraint coincident L18.end A3.centre
  constraint coincident L14 L24.end
  constraint perpendicular L14 L24
  constraint coincident L10 L25.end
  constraint perpendicular L10 L25
  constraint coincident L18.start A4.centre
  measures "d224" distance of L13.end L14.end
  measures "d225" distance of L14.end L15.end
  measures "d226" distance of L15.end L16.end
  measures "d228" distance of L18.start L18.end
  measures "d229" distance of L16.end L19.end
  measures "d230" distance of L14.end L20.end
  measures "d231" distance of L14.end L22.end
  measures "d232" diameter of A1
  measures "d233" diameter of A2
  measures "d234" diameter of A3
  measures "d236" diameter of A4
extrude "Extrude1''" add sketch "Sketch1 (3)" along normal blind 2 separate body contours L0 L1 L2 L3 L4 L5 L6 L7 L8 L9 L10 L25 L29 L30 L31 L32 | L0 L1 L2 L3 L4 L5 L6 L14 L15 L16 L17 L21 L22 A1 L24 L29 L30 L31 L32 | L14 L15 L20 L21 L22 L23 A1 makes body 3 in component "BottomLid"
sketch "Sketch1 (4)" plane through (0, -4, 0) normal (0, -1, 0) x (1, 0, 0) in component "TopLid"
  circle A0 centre (12, -41.75) radius 0.95
  line L0 (28, -32.1519) -> (58, -32.1519)
  arc A1 (58, -48.3481) -> (58, -32.1519) centre (58, -40.25) ccw
  line L1 (58, -48.3481) -> (28, -48.3481)
  arc A2 (28, -32.1519) -> (28, -48.3481) centre (28, -40.25) ccw
  line L2 (67, -19) -> (67, -30)
  line L3 (2, -30) -> (2, -19)
  line L4 (2, -19) -> (4.5, -19)
  line L5 (4.5, -19) -> (4.5, -11)
  line L6 (4.5, -11) -> (2, -11)
  line L7 (2, -11) -> (2, 0)
  line L8 (2, 0) -> (0, 0)
  line L9 (0, 0) -> (0, -51.75)
  line L10 (0, -51.75) -> (69, -51.75)
  line L11 (69, -51.75) -> (69, 0)
  line L12 (69, 0) -> (67, 0)
  line L13 (67, 0) -> (67, -11)
  line L14 (67, -11) -> (64.5, -11)
  line L15 (64.5, -11) -> (64.5, -19)
  line L16 (64.5, -19) -> (67, -19)
  circle A3 centre (2.25, -15) radius 0.95
  circle A4 centre (66.75, -15) radius 0.95
  line L17 (0, 0) -> (0, 22.5)
  line L18 (0, 22.5) -> (69, 22.5)
  line L19 (69, 22.5) -> (69, 0)
  line L20 (69, 0) -> (0, 0)
  line L21 (0, 0) -> (0, 22.5)
  line L22 (0, 0) -> (0, 10)
  line L23 (0, 10) -> (2.25, 10)
  line L24 (2.25, 10) -> (66.75, 10)
  circle A5 centre (2.25, 10) radius 0.95
  circle A6 centre (66.75, 10) radius 0.95
  line L25 (67, -30) -> (2, -30)
  dimension "d239" = 22.5
  dimension "d240" = 10
  dimension "d241" = 2.25
  dimension "d242" = 64.5
  dimension "d243" = 1.9
  dimension "d244" = 1.9
  constraint coincident L8.end L9.start
  constraint perpendicular L8 L17
  constraint horizontal L18
  constraint vertical L19
  constraint horizontal L20
  constraint vertical L21
  constraint coincident L11.end L12.start
  constraint perpendicular L8 L22
  constraint perpendicular L21 L23
  constraint parallel L23 L24
  constraint coincident L23.end L24.start
  constraint coincident L24.end A6.centre
  measures "d239" distance of L8.end L17.end
  measures "d240" distance of L8.end L22.end
  measures "d241" distance of L22.end L23.end
  measures "d242" distance of L23.end L24.end
  measures "d243" diameter of A5
  measures "d244" diameter of A6
extrude "Extrude1'''" add sketch "Sketch1 (4)" along normal blind 2 separate body makes body 4 in component "TopLid"
sketch "Sketch7 (2)" plane through (0, 0, -49.75) normal (0, 0, 1) x (1, 0, 0) in component "TopPart"
  arc A0 (67, 8.5) -> (65.5, 10) centre (65.5, 8.5) ccw
  line L0 (65.5, 10) -> (65.5, 11)
  line L1 (65.5, 11) -> (3.5, 11)
  line L2 (3.5, 11) -> (3.5, 10)
  arc A1 (3.5, 10) -> (2, 8.5) centre (3.5, 8.5) ccw
  line L3 (2, 8.5) -> (2, 0.5)
  line L4 (2, 0.5) -> (67, 0.5)
  line L5 (67, 0.5) -> (67, 8.5)
  line L6 (2, 0.5) -> (10, 0.5)
  line L7 (10, 0.5) -> (10, 5.25)
  line L8 (10, 5.25) -> (2, 5.25)
  line L9 (2, 5.25) -> (2, 0.5)
  circle A2 centre (10, 5.25) radius 3.5
  dimension "d247" = 8
  dimension "d248" = 4.75
  dimension "d249" = 7
  constraint horizontal L6
  constraint vertical L7
  constraint horizontal L8
  constraint vertical L9
  constraint coincident L3.end L4.start
  constraint coincident L7.end L8.start
  measures "d247" distance of L3.end L6.end
  measures "d248" distance of L3.end L8.end
  measures "d249" diameter of A2
extrude "Extrude13'" cut sketch "Sketch7 (2)" against normal blind 2 contours L7 L8 A2 | L7 L8 A2 bodies 2 in component "TopPart"
sketch "Sketch2 (4)" plane through (0, -4, 0) normal (0, 1, 0) x (-1, 0, 0) in component "BottomLid"
  circle A0 centre (-41, 75) radius 0.95
  circle A1 centre (-3, 82) radius 0.95
  circle A2 centre (-66, 82) radius 0.95
  circle A3 centre (-66.75, 30) radius 0.95
  line L0 (-69, 90) -> (-69, 22.5)
  line L1 (-69, 22.5) -> (0, 22.5)
  line L2 (0, 22.5) -> (0, 90)
  line L3 (0, 90) -> (-28, 90)
  line L4 (-28, 90) -> (-28, 80)
  line L5 (-28, 80) -> (-41, 80)
  line L6 (-41, 80) -> (-41, 90)
  line L7 (-41, 90) -> (-69, 90)
  line L8 (-28, 80) -> (-30.5, 80)
  line L9 (-30.5, 80) -> (-38.5, 80)
  line L10 (-38.5, 80) -> (-38.5, 70)
  line L11 (-38.5, 70) -> (-30.5, 70)
  line L12 (-30.5, 70) -> (-30.5, 80)
  circle A4 centre (-2.25, 30) radius 0.95
  dimension "d252" = 2.5
  dimension "d253" = 8
  dimension "d254" = 10
  constraint coincident L4.end L5.start
  constraint perpendicular L4 L8
  constraint horizontal L9
  constraint vertical L10
  constraint horizontal L11
  constraint vertical L12
  measures "d252" distance of L4.end L8.end
  measures "d253" distance of L8.end L9.end
  measures "d254" distance of L8.end L11.end
extrude "Extrude2''" cut sketch "Sketch2 (4)" against normal blind 2 contours L5 L9 L10 L11 L12 bodies 3 in component "BottomLid"
sketch "Sketch3 (3)" plane through (0, -4, 0) normal (0, 1, 0) x (-1, 0, 0) in component "BottomLid"
  line L0 (-30.5, 80) -> (-30.5, 70)
  line L1 (-30.5, 70) -> (-38.5, 70)
  line L2 (-38.5, 70) -> (-38.5, 80)
  line L3 (-38.5, 80) -> (-41, 80)
  line L4 (-41, 80) -> (-41, 90)
  line L5 (-41, 90) -> (-69, 90)
  line L6 (-69, 90) -> (-69, 22.5)
  line L7 (-69, 22.5) -> (0, 22.5)
  line L8 (0, 22.5) -> (0, 90)
  line L9 (0, 90) -> (-28, 90)
  line L10 (-28, 90) -> (-28, 80)
  line L11 (-28, 80) -> (-30.5, 80)
  circle A0 centre (-66.75, 30) radius 0.95
  circle A1 centre (-66, 82) radius 0.95
  circle A2 centre (-3, 82) radius 0.95
  circle A3 centre (-41, 75) radius 0.95
  line L12 (-69, 90) -> (-58.1, 90)
  line L13 (-58.1, 90) -> (-48.9, 90)
  line L14 (-48.9, 90) -> (-48.9, 88)
  line L15 (-48.9, 88) -> (-58.1, 88)
  line L16 (-58.1, 88) -> (-58.1, 90)
  line L17 (-58.1, 88) -> (-64, 88)
  line L18 (-64, 88) -> (-43, 88)
  line L19 (-43, 88) -> (-43, 61)
  line L20 (-43, 61) -> (-64, 61)
  line L21 (-64, 61) -> (-64, 88)
  line L22 (-43, 61) -> (-20, 61)
  line L23 (-20, 61) -> (-20, 65)
  line L24 (-20, 65) -> (-43, 65)
  line L25 (-43, 65) -> (-43, 61)
  line L26 (-64, 61) -> (-67, 61)
  line L27 (-67, 61) -> (-67, 65)
  line L28 (-67, 65) -> (-64, 65)
  line L29 (-64, 65) -> (-64, 61)
  circle A4 centre (-2.25, 30) radius 0.95
  line L30 (-67, 61) -> (-64, 61)
  line L31 (-64, 61) -> (-64, 60)
  line L32 (-64, 60) -> (-67, 60)
  line L33 (-67, 60) -> (-67, 61)
  line L34 (-67, 60) -> (-52, 60)
  line L35 (-52, 60) -> (-52, 55)
  line L36 (-52, 55) -> (-67, 55)
  line L37 (-67, 55) -> (-67, 60)
  dimension "d257" = 10.9
  dimension "d258" = 9.2
  dimension "d259" = 2
  dimension "d260" = 5.9
  dimension "d261" = 21
  dimension "d262" = 27
  dimension "d265" = 23
  dimension "d266" = 4
  dimension "d267" = 3
  dimension "d268" = 4
  dimension "d283" = 3
  dimension "d284" = 1
  dimension "d285" = 15
  dimension "d286" = 5
  constraint coincident L5.end L6.start
  constraint perpendicular L6 L12
  constraint horizontal L13
  constraint vertical L14
  constraint horizontal L15
  constraint vertical L16
  constraint perpendicular L16 L17
  constraint horizontal L18
  constraint vertical L19
  constraint horizontal L20
  constraint vertical L21
  constraint horizontal L22
  constraint vertical L23
  constraint horizontal L24
  constraint vertical L25
  constraint horizontal L26
  constraint vertical L27
  constraint horizontal L28
  constraint vertical L29
  constraint horizontal L30
  constraint vertical L31
  constraint horizontal L32
  constraint vertical L33
  constraint horizontal L34
  constraint vertical L35
  constraint horizontal L36
  constraint vertical L37
  measures "d257" distance of L5.end L12.end
  measures "d258" distance of L12.end L13.end
  measures "d259" distance of L12.end L15.end
  measures "d260" distance of L15.end L17.end
  measures "d261" distance of L17.end L18.end
  measures "d262" distance of L17.end L20.end
  measures "d265" distance of L19.end L22.end
  measures "d266" distance of L19.end L24.end
  measures "d267" distance of L20.end L26.end
  measures "d268" distance of L20.end L28.end
  measures "d283" distance of L26.end L20.end
  measures "d284" distance of L26.end L32.end
  measures "d285" distance of L32.end L34.end
  measures "d286" distance of L32.end L36.end
extrude "Extrude3''" cut sketch "Sketch3 (3)" against normal blind 1.5 contours L5 L13 L14 L15 L16 L18 | L15 L17 L18 L19 L20 L21 L25 L29 | L19 L22 L23 L24 L25 | L21 L26 L27 L28 L29 L30 | L26 L30 L31 L32 L33 L34 | L32 L34 L35 L36 L37 bodies 3 in component "BottomLid"
sketch "Sketch15" plane through (67, 0, 0) normal (-1, 0, 0) x (0, 0, 1) in component "BottomPart"
  line L0 (80, 8.5) -> (23.5, 8.5)
  line L1 (23.5, 8.5) -> (23.5, 2.25)
  line L2 (23.5, 2.25) -> (0, 2.25)
  line L3 (0, 2.25) -> (0, 0.5)
  line L4 (0, 0.5) -> (80, 0.5)
  line L5 (80, 0.5) -> (80, 8.5)
  line L6 (80, 0.5) -> (52, 0.5)
  line L7 (52, 0.5) -> (52, 2.25)
  line L8 (52, 2.25) -> (80, 2.25)
  line L9 (80, 2.25) -> (80, 0.5)
  line L10 (52, 2.25) -> (45, 2.25)
  line L11 (45, 2.25) -> (59, 2.25)
  line L12 (59, 2.25) -> (59, 8.25)
  line L13 (59, 8.25) -> (45, 8.25)
  line L14 (45, 8.25) -> (45, 2.25)
  dimension "d269" = 28
  dimension "d270" = 1.75
  dimension "d271" = 7
  dimension "d272" = 14
  dimension "d273" = 6
  constraint horizontal L6
  constraint vertical L7
  constraint horizontal L8
  constraint vertical L9
  constraint coincident L4.end L5.start
  constraint perpendicular L7 L10
  constraint horizontal L11
  constraint vertical L12
  constraint horizontal L13
  constraint vertical L14
  measures "d269" distance of L4.end L6.end
  measures "d270" distance of L4.end L8.end
  measures "d271" distance of L7.end L10.end
  measures "d272" distance of L10.end L11.end
  measures "d273" distance of L10.end L13.end
extrude "Extrude23" cut sketch "Sketch15" against normal blind 2 contours L8 L10 L11 L12 L13 L14 bodies 1 in component "BottomPart"
extrude "Extrude14'" cut 1 faces at (23.6667, -2.6667, -30) along direction (0, 0, -1) blind 1.5 on bodies 2 bodies 2 in component "TopPart"
sketch "Sketch16" plane through (0, 0, 0) normal (0, -1, 0) x (1, 0, 0) in component "BottomPart"
  line L0 (64.5, 34) -> (67, 34)
  line L1 (67, 34) -> (67, 65)
  line L2 (67, 65) -> (64, 65)
  line L3 (64, 65) -> (64, 88)
  line L4 (64, 88) -> (43, 88)
  line L5 (43, 88) -> (43, 65)
  line L6 (43, 65) -> (39, 65)
  line L7 (39, 65) -> (39, 78)
  line L8 (39, 78) -> (38.5, 78)
  line L9 (38.5, 78) -> (38.5, 80)
  line L10 (38.5, 80) -> (30.5, 80)
  line L11 (30.5, 80) -> (30.5, 78)
  line L12 (30.5, 78) -> (20, 78)
  line L13 (20, 78) -> (20, 61)
  line L14 (20, 61) -> (64, 61)
  line L15 (64, 61) -> (64, 60)
  line L16 (64, 60) -> (2, 60)
  line L17 (2, 60) -> (2, 34)
  line L18 (2, 34) -> (4.5, 34)
  line L19 (4.5, 34) -> (4.5, 26)
  line L20 (4.5, 26) -> (2, 26)
  line L21 (2, 26) -> (2, 14)
  line L22 (2, 14) -> (4.5, 14)
  line L23 (4.5, 14) -> (4.5, 6)
  line L24 (4.5, 6) -> (2, 6)
  line L25 (2, 6) -> (2, 0)
  line L26 (2, 0) -> (67, 0)
  line L27 (67, 0) -> (67, 6)
  line L28 (67, 6) -> (64.5, 6)
  line L29 (64.5, 6) -> (64.5, 14)
  line L30 (64.5, 14) -> (67, 14)
  line L31 (67, 14) -> (67, 26)
  line L32 (67, 26) -> (64.5, 26)
  line L33 (64.5, 26) -> (64.5, 34)
  line L34 (64, 61) -> (62, 61)
  line L35 (62, 61) -> (54, 61)
  line L36 (54, 61) -> (54, 62.5)
  line L37 (54, 62.5) -> (62, 62.5)
  line L38 (62, 62.5) -> (62, 61)
  dimension "d278" = 2
  dimension "d279" = 8
  dimension "d280" = 1.5
  constraint coincident L14.end L15.start
  constraint perpendicular L15 L34
  constraint horizontal L35
  constraint vertical L36
  constraint horizontal L37
  constraint vertical L38
  measures "d278" distance of L14.end L34.end
  measures "d279" distance of L34.end L35.end
  measures "d280" distance of L34.end L37.end
extrude "Extrude24" add sketch "Sketch16" along normal blind 4 contours L14 L35 L36 L37 L38 bodies 1 in component "BottomPart"